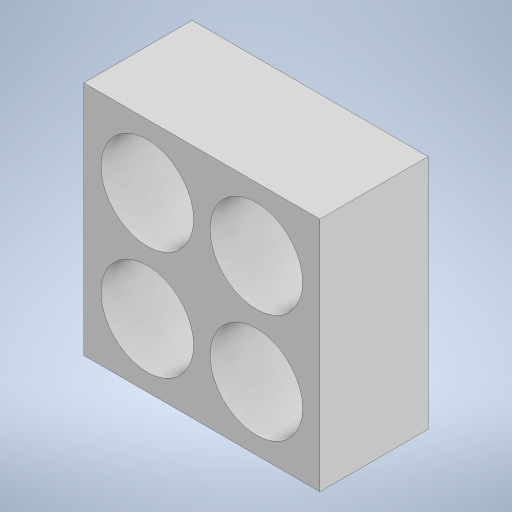
# Autodesk Inventor part: Cell Grid (2x2)
Saved by Autodesk Inventor 2024 (Build 280153000, 153)
## iProperties
Created: 2024-10-10
Part Number: Cell Grid (2x2)
Material: Generic
Document SubType Name: Modeling
Designer: v
Density: 1 g/cm^3
Appearance: Default
Author: v
Autodesk Inventor part; units mm, degrees
ref_plane "YZ Plane" through (0, 0, 0) normal (1, 0, 0) x (0, 1, 0)
ref_plane "XZ Plane" through (0, 0, 0) normal (0, 1, 0) x (-1, 0, 0)
ref_plane "XY Plane" through (0, 0, 0) normal (0, 0, 1) x (1, 0, 0)
sketch "Sketch1" plane through (0, 0, 0) normal (0, 0, 1) x (1, 0, 0)
  line L0 (-35.6669, 19.4148) -> (19.7051, 19.4148)
  line L1 (19.7051, 19.4148) -> (19.7051, -35.9572)
  line L2 (19.7051, -35.9572) -> (-35.6669, -35.9572)
  line L3 (-35.6669, -35.9572) -> (-35.6669, 19.4148)
  circle A0 centre (4.8029, 4.5126) radius 10.8585
  circle A1 centre (-20.7672, 4.5126) radius 10.8585
  circle A2 centre (4.8029, -21.0575) radius 10.8585
  circle A3 centre (-20.7672, -21.0575) radius 10.8585
  dimension "d3" = 21.717
  dimension "d6" = 14.9022
  dimension "d7" = 14.9022
  dimension "d12" = 25.5702
  dimension "d15" = 25.5702
  dimension "d20" = 14.8996
  dimension "d21" = 14.8996
  constraints: 8 end point, 4 centre point, 2 horizontal, 2 parallel, 1 perpendicular, 1 vertical, 6 other
  measures "d3" diameter of A0
  measures "d6" distance from line of L1 A0.centre
  measures "d7" distance from line of L0 A0.centre
  measures "d12" distance of A0.centre A1.centre
  measures "d15" distance of A0.centre A2.centre
  measures "d20" distance from line of L2 A3.centre
  measures "d21" distance from line of L3 A3.centre
extrude "Extrusion1" add sketch "Sketch1" along normal blind 25.4
equation "\"d15\" = d12"
body "Solid1"
